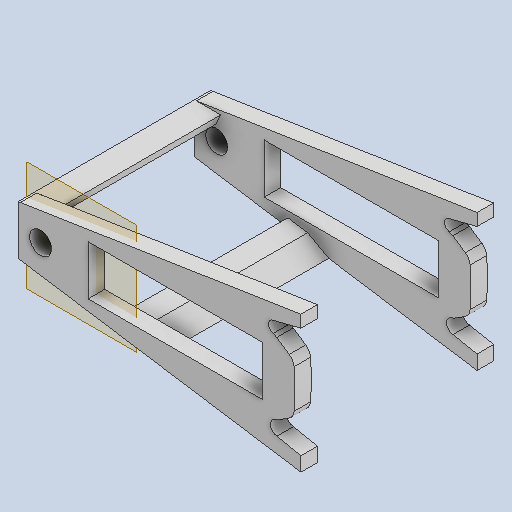
# Autodesk Inventor part: Cage
Saved by Autodesk Inventor 2025 (Build 290162000, 162)
## iProperties
Created: 2025-08-05
Part Number: Cage
Material: Generic
Document SubType Name: Modeling
Designer: Pravoslav
Density: 1 g/cm^3
Appearance: Default
Author: Pravoslav
Autodesk Inventor part; units mm, degrees
ref_plane "YZ Plane" through (0, 0, 0) normal (1, 0, 0) x (0, 1, 0)
ref_plane "XZ Plane" through (0, 0, 0) normal (0, 1, 0) x (-1, 0, 0)
ref_plane "Work Plane1" through (0, 0, 16) normal (0, 0, 1) x (1, 0, 0)
sketch "Sketch1" plane through (0, 0, 16) normal (0, 0, 1) x (1, 0, 0)
  circle A0 centre (-6, 0) radius 2
  line L0 (-10.0224, 4.5) -> (39.9776, 4.5)
  line L1 (39.9776, 4.5) -> (39.9776, -4.5)
  line L2 (39.9776, -4.5) -> (-10.0224, -4.5)
  line L3 (-10.0224, -4.5) -> (-10.0224, 4.5)
  line L4 (39.9776, 4.5) -> (36.5254, 6.8216)
  line L5 (39.9776, -4.5) -> (36.9512, -6.4067)
  arc A1 (36.5254, 9.0045) -> (36.5254, 6.8216) centre (36.4895, 7.9131) ccw
  arc A2 (36.9512, -6.4067) -> (36.9512, -8.9625) centre (37.0427, -7.6846) ccw
  line L6 (36.5254, 9.0045) -> (41.3206, 10.2245)
  line L7 (41.3206, 10.2245) -> (41.3206, 12.4243)
  line L8 (41.3206, 12.4243) -> (-9.6772, 4.5)
  line L9 (36.9512, -8.9625) -> (41.3206, -9.8433)
  line L10 (41.3206, -9.8433) -> (41.3206, -12.4334)
  line L11 (41.3206, -12.4334) -> (-10.0224, -4.5)
  circle A3 centre (-6, 0) radius 46.1973
  line L12 (2.6468, -4.5) -> (34.2776, -4.5)
  line L13 (34.2776, -4.5) -> (34.2776, 4.5)
  line L14 (34.2776, 4.5) -> (2.6468, 4.5)
  line L15 (2.6468, 4.5) -> (2.6468, -4.5)
  point P0 (0, 0)
  point P1 (2.6468, 4.5)
  dimension "d1" = 4
  dimension "d2" = 50
  dimension "d3" = 9
  dimension "d4" = 4.5
  dimension "d5" = 6
  constraints: 32 end point, 5 point on line, 4 parallel, 4 point on circle, 3 centre point, 2 horizontal, 2 perpendicular, 1 coincident, 1 vertical, 3 other
  measures "d1" diameter of A0
  measures "d2" distance of L1.end L2.end
  measures "d3" distance of L0.end L1.end
  measures "d4" distance from line of L0 point (0, 0)
  measures "d5" distance of point (0, 0) A0.centre
extrude "Extrusion1" add sketch "Sketch1" along normal mid plane 3 contours L0 L15 L2 L3 | L8 A3 L6 A1 L4 L0 | L2 L5 A2 L9 A3 L11 | L8 L7 L6 A3 | A3 L9 L10 L11 | L0 L1 L2 L13 | A3 L1
mirror "Mirror1" about plane through (0, 0, 0) normal (0, 0, 1) of "Extrusion1"
fillet "Fillet1" radius 2 8 edges at (39.9776, -4.5, -16) (39.9776, 4.5, -16) (39.9776, -4.5, 16) (39.9776, 4.5, 16) (36.5254, 6.8216, 16) (36.9512, -6.4067, 16) (36.9512, -6.4067, -16) (36.5254, 6.8216, -16)
sketch "Sketch2" plane through (-10.0224, -4.5, -14.5) normal (0, 0, 1) x (1, 0, 0)
  line L0 (0, 9) -> (0, 0) projected
  line L1 (10.0224, 7.1192) -> (0, 7.1192)
  line L2 (0, 7.1192) -> (0, 9)
  line L3 (0, 9) -> (10.0224, 9)
  line L4 (10.0224, 9) -> (10.0224, 7.1192)
  line L5 (0, 0) -> (51.3431, -7.9334) projected
  line L6 (24.3876, -3.7683) -> (16.7368, -2.5861)
  line L7 (16.9636, -1.0923) -> (24.6183, -2.2751)
  line L8 (24.6183, -2.2751) -> (24.3876, -3.7683)
  line L9 (16.7368, -2.5861) -> (16.9877, -0.9624)
  line L10 (16.9877, -0.9624) -> (16.7368, -2.5861)
  line L11 (24.3876, -3.7683) -> (16.7368, -2.5861)
  line L12 (3.8915, 7.1192) -> (4.7568, 9)
  line L13 (24.3876, -3.7683) -> (20.5622, -1.6484)
  point P0 (10.0224, 4.5)
  point P1 (16.9675, -1.0929)
  constraints: 24 end point, 5 point on line, 3 parallel, 2 collinear, 2 perpendicular, 1 horizontal
extrude "Extrusion2" add sketch "Sketch2" along normal up to surface (29 mm away) contours L3 L12 L1 L0 | L9 L7 L13 L5
body "Solid1"
